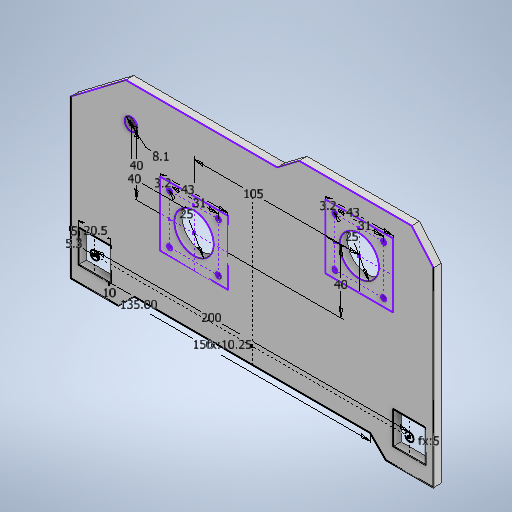
# Autodesk Inventor part: Motor-Side
Saved by Autodesk Inventor 2025.3 (Build 293356030, 356C)
## iProperties
Created: 2025-09-01
Part Number: Motor-Side
Material: Generic
Document SubType Name: Modeling
Designer: tvoko
Density: 1 g/cm^3
Appearance: Default
Author: tvoko
Autodesk Inventor part; units mm, degrees
ref_plane "YZ Plane" through (0, 0, 0) normal (1, 0, 0) x (0, 1, 0)
ref_plane "XZ Plane" through (0, 0, 0) normal (0, 1, 0) x (-1, 0, 0)
ref_plane "XY Plane" through (0, 0, 0) normal (0, 0, 1) x (1, 0, 0)
sketch "Sketch1" plane through (0, 0, 0) normal (0, 0, 1) x (1, 0, 0)
  line L0 (-20.5, 20.5) -> (0, 20.5)
  line L1 (0, 20.5) -> (0, 0)
  line L2 (0, 0) -> (-20.5, 0)
  line L3 (-20.5, 0) -> (-20.5, 20.5)
  line L4 (-25.5, -10) -> (4.75, -10)
  line L5 (4.75, -10) -> (14.75, 0)
  line L6 (14.75, 0) -> (164.75, 0)
  line L7 (164.75, 0) -> (174.75, -10)
  line L8 (174.75, -10) -> (205, -10)
  line L9 (205, -10) -> (205, 110.98)
  line L10 (-25.5, -10) -> (-25.5, 90.0042)
  line L11 (89.75, 0) -> (89.75, 91.5139) construction
  line L12 (-10.25, 20.5) -> (-10.25, 0) construction
  line L13 (179.5, 20.5) -> (200, 20.5)
  line L14 (200, 20.5) -> (200, 0)
  line L15 (200, 0) -> (179.5, 0)
  line L16 (179.5, 0) -> (179.5, 20.5)
  line L17 (189.75, 20.5) -> (189.75, 0) construction
  line L18 (-10.25, 10.25) -> (189.75, 10.25) construction
  line L19 (37.3718, 69.4481) -> (68.3718, 69.4481) construction
  line L20 (68.3718, 69.4481) -> (68.3718, 38.4481) construction
  line L21 (68.3718, 38.4481) -> (37.3718, 38.4481) construction
  line L22 (37.3718, 38.4481) -> (37.3718, 69.4481) construction
  line L23 (31.3718, 74.3149) -> (74.3718, 74.3149)
  line L24 (74.3718, 74.3149) -> (74.3718, 33.5812)
  line L25 (74.3718, 33.5812) -> (31.3718, 33.5812)
  line L26 (31.3718, 33.5812) -> (31.3718, 74.3149)
  line L27 (52.8718, 74.3149) -> (52.8718, 33.5812) construction
  line L28 (31.3718, 53.9481) -> (74.3718, 53.9481) construction
  circle A0 centre (37.3718, 69.4481) radius 1.6
  circle A1 centre (68.3718, 69.4481) radius 1.6
  circle A2 centre (68.3718, 38.4481) radius 1.6
  circle A3 centre (37.3718, 38.4481) radius 1.6
  circle A4 centre (52.8718, 53.9481) radius 12.5
  line L29 (142.3718, 109.4481) -> (173.3718, 109.4481) construction
  line L30 (173.3718, 109.4481) -> (173.3718, 78.4481) construction
  line L31 (173.3718, 78.4481) -> (142.3718, 78.4481) construction
  line L32 (142.3718, 78.4481) -> (142.3718, 109.4481) construction
  line L33 (136.3718, 114.3149) -> (179.3718, 114.3149)
  line L34 (179.3718, 114.3149) -> (179.3718, 73.5812)
  line L35 (179.3718, 73.5812) -> (136.3718, 73.5812)
  line L36 (136.3718, 73.5812) -> (136.3718, 114.3149)
  line L37 (157.8718, 114.3149) -> (157.8718, 73.5812) construction
  line L38 (136.3718, 93.9481) -> (179.3718, 93.9481) construction
  circle A5 centre (142.3718, 109.4481) radius 1.6
  circle A6 centre (173.3718, 109.4481) radius 1.6
  circle A7 centre (173.3718, 78.4481) radius 1.6
  circle A8 centre (142.3718, 78.4481) radius 1.6
  circle A9 centre (157.8718, 93.9481) radius 12.5
  circle A10 centre (-10.25, 10.25) radius 2.65
  circle A11 centre (189.75, 10.25) radius 2.65
  circle A12 centre (12.8718, 93.9481) radius 4.05
  line L39 (205, 110.98) -> (191.1506, 127.1705)
  line L40 (191.1506, 127.1705) -> (119.6721, 127.1705)
  line L41 (119.6721, 127.1705) -> (105.6894, 116.5684)
  line L42 (105.6894, 116.5684) -> (9.5346, 116.5684)
  line L43 (9.5346, 116.5684) -> (-25.5, 90.0042)
  point P0 (89.75, 10.25)
  point P1 (52.8718, 69.4481)
  point P2 (37.3718, 53.9481)
  point P3 (157.8718, 109.4481)
  point P4 (142.3718, 93.9481)
  dimension "d0" = 20.5
  dimension "d1" = 200
  dimension "d2" = 5
  dimension "d3" = 5
  dimension "d4" = 10
  dimension "d5" = 10.25
  dimension "d6" = 135
  dimension "d7" = 150
  dimension "d8" = 31
  dimension "d9" = 43
  dimension "d10" = 3.2
  dimension "d11" = 25
  dimension "d12" = 31
  dimension "d13" = 43
  dimension "d14" = 3.2
  dimension "d15" = 25
  dimension "d16" = 5.3
  dimension "d21" = 40
  dimension "d22" = 105
  dimension "d23" = 8.1
  dimension "d24" = 40
  dimension "d25" = 40
  constraints: 88 end point, 22 midpoint, 15 parallel, 13 centre point, 10 coincident, 9 perpendicular, 8 horizontal, 7 equal radius, 7 point on line, 5 equal length, 2 vertical
  measures "d0" distance of L0.start L0.end
  measures "d1" distance of L18.start L18.end
  measures "d2" distance between parallel lines of L10 L3
  measures "d3" distance between parallel lines of L14 L9
  measures "d4" distance between parallel lines of L4 L6
  measures "d5" distance between parallel lines of L6 L18
  measures "d6" angle of L6 L5
  measures "d7" distance of L5.end L6.end
  measures "d8" distance of L19.start L19.end
  measures "d9" distance of L23.start L23.end
  measures "d10" diameter of A0
  measures "d11" diameter of A4
  measures "d12" distance of L29.start L30.start
  measures "d13" distance of L33.start L34.start
  measures "d14" diameter of A5
  measures "d15" diameter of A9
  measures "d16" diameter of A10
  measures "d21" distance between parallel lines of L28 L38
  measures "d22" distance between parallel lines of L27 L37
  measures "d23" diameter of A12
  measures "d24" distance from line of A12.centre L27
  measures "d25" distance from line of A12.centre L28
extrude "Extrusion1" add sketch "Sketch1" against normal blind 5 contours L10 L43 L42 L41 L40 L39 L9 L8 L7 L6 L5 L4 | L23 L24 L25 L26 | L33 L34 L35 L36
equation "\"d3\" = d2"
equation "\"d5\" = 0.5 * d0"
body "Solid1"
